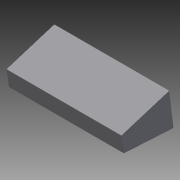
# Autodesk Inventor part: Prow
Saved by Autodesk Inventor 2015 (Build 190159000, 159)
## iProperties
Created: 2016-01-19
Part Number: Prow
Material: Generic
Document SubType Name: Modeling
Designer: sethbattis
Density: 1 g/cm^3
Appearance: Default
Author: sethbattis
Autodesk Inventor part; units mm, degrees
ref_plane "YZ Plane" through (0, 0, 0) normal (1, 0, 0) x (0, 1, 0)
ref_plane "XZ Plane" through (0, 0, 0) normal (0, 1, 0) x (-1, 0, 0)
ref_plane "XY Plane" through (0, 0, 0) normal (0, 0, 1) x (1, 0, 0)
sketch "Sketch4" plane through (0, 0, 0) normal (1, 0, 0) x (0, 1, 0)
  line L0 (0, 0) -> (0, -196.85) construction
  line L1 (0, -196.85) -> (127, -196.85) construction
  line L2 (127, -196.85) -> (166.8671, 0) construction
  line L3 (166.8671, 0) -> (304.8, 0) construction
  line L4 (304.8, 0) -> (304.8, -196.85) construction
  line L5 (-649.2599, 0) -> (1006.3094, 0) construction
  line L6 (0, -1144.2085) -> (0, 1442.3512) construction
  line L7 (101.6, -275.7538) -> (101.6, 0) construction
  line L8 (304.8, 0) -> (177.8, 0) construction
  line L9 (177.8, 0) -> (177.8, 50.8) construction
  line L10 (209.55, 82.55) -> (273.05, 82.55) construction
  line L11 (304.8, 50.8) -> (304.8, 0) construction
  arc A0 (304.8, 50.8) -> (273.05, 82.55) centre (273.05, 50.8) ccw construction
  arc A1 (209.55, 82.55) -> (177.8, 50.8) centre (209.55, 50.8) ccw construction
  circle A2 centre (127, -196.85) radius 127 construction
  line L12 (127, -196.85) -> (165.1, -196.85) construction
  circle A3 centre (165.1, -196.85) radius 301.905 construction
  line L13 (0, 0) -> (0, 381) construction
  line L14 (0, 381) -> (769.7995, 381) construction
  circle A4 centre (165.1, -196.85) radius 577.85 construction
  line L15 (97.7502, 99.0287) -> (284.0621, 122.0519)
  line L16 (128.0743, 102.776) -> (165.1, -196.85) construction
  line L17 (0, -127) -> (0, 381) construction
  line L18 (0, 381) -> (76.2, 381) construction
  line L19 (76.2, 381) -> (76.2, 168.1213) construction
  line L20 (76.2, 168.1213) -> (0, -127) construction
  line L21 (76.2, 381) -> (203.2, 381) construction
  line L22 (203.2, 381) -> (203.2, 430.7829)
  line L23 (203.2, 381) -> (284.0621, 122.0519)
  line L24 (203.2, 381) -> (113.307, 367.5826)
  line L25 (113.307, 367.5826) -> (97.7502, 99.0287)
  line L26 (76.2, 168.1213) -> (76.2, 777.7213) construction
  line L27 (76.2, 777.7213) -> (0, 1072.8427) construction
  line L28 (76.2, 472.9213) -> (171.45, 472.9213) construction
  circle A5 centre (171.45, 472.9213) radius 25.4 construction
  line L29 (87.8983, 768.5119) -> (76.2, 763.5683)
  line L30 (76.2, 763.5683) -> (313.4933, 202.0488) construction
  line L31 (313.4933, 202.0488) -> (325.1916, 206.9925) construction
  line L32 (325.1916, 206.9925) -> (87.8983, 768.5119) construction
  circle A6 centre (171.45, 472.9213) radius 25.4 construction
  line L33 (194.8466, 482.8086) -> (148.0534, 463.0341) construction
  line L34 (250.4975, 95.1372) -> (422.8203, 20.6587) construction
  line L35 (422.8203, 20.6587) -> (484.1983, 284.904) construction
  line L36 (484.1983, 284.904) -> (399.8857, 318.8477) construction
  line L37 (399.8857, 318.8477) -> (250.4975, 95.1372) construction
  line L38 (399.8857, 318.8477) -> (422.8203, 20.6587) construction
  line L39 (484.1983, 284.904) -> (250.4975, 95.1372) construction
  line L40 (203.2, 381) -> (97.7502, 99.0287) construction
  line L41 (113.307, 367.5826) -> (284.0621, 122.0519) construction
  point P0 (177.8, 82.55)
  point P1 (304.8, 82.55)
  dimension "d44" = 196.85
  dimension "d45" = 127
  dimension "d46" = 304.8
  dimension "d47" = 101.6
  dimension "d48" = 127
  dimension "d50" = 31.75
  dimension "d51" = 254
  dimension "d53" = 381
  dimension "d54" = 508
  dimension "d55" = 76.2
  dimension "d56" = 304.8
  dimension "d57" = 127
  dimension "d58" = 38.1
  dimension "d59" = 609.6
  dimension "d60" = 304.8
  dimension "d61" = 95.25
  dimension "d62" = 50.8
  dimension "d65" = 609.6
  dimension "d66" = 50.8
  dimension "d67" = 11.6983
  dimension "d68" = 12.7
  dimension "d74" = 82.55
  constraints: 80 end point, 13 point on line, 9 horizontal, 9 tangent, 7 equal length, 6 centre point, 6 point on circle, 4 coincident, 4 midpoint, 4 parallel, 4 perpendicular, 4 vertical, 2 collinear, 1 concentric, 1 equal radius, 1 symmetric about line, 4 other
  measures "d44" distance of L0.start L0.end
  measures "d45" distance of L0.end L1.end
  measures "d46" distance between parallel lines of L0 L4
  measures "d47" distance between parallel lines of L0 L7
  measures "d48" distance of point (177.8, 82.55) point (304.8, 82.55)
  measures "d50" radius of A0
  measures "d51" diameter of A2
  measures "d53" distance of L0.start L13.end
  measures "d54" distance of L17.start L17.end
  measures "d55" distance of L17.end L18.end
  measures "d56" distance of L19.end L17.start
  measures "d57" distance of L18.end L21.end
  measures "d58" distance of L12.start L12.end
  measures "d59" distance of L19.end L26.end
  measures "d60" distance of L26.end L27.end
  measures "d61" distance of L28.start L28.end
  measures "d62" diameter of A5
  measures "d65" distance of L30.end L29.end
  measures "d66" diameter of A6
  measures "d67" horizontal distance of L29.start L29.end
  measures "d68" distance of L29.start L29.end
  measures "d74" distance between parallel lines of L3 L10
extrude "Extrusion3" add sketch "Sketch4" along normal blind 622.3
body "Solid2"
